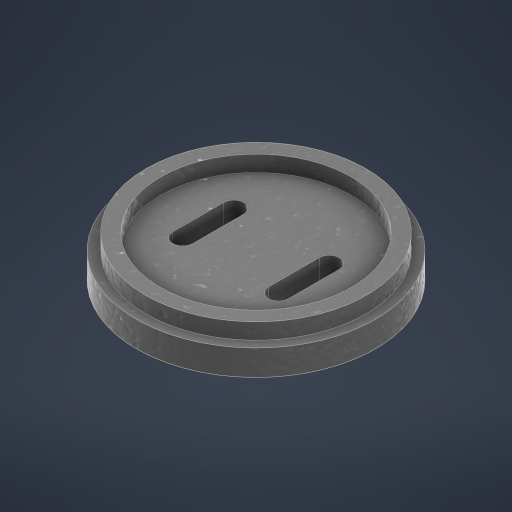
# Autodesk Inventor part: bay_bottom
Saved by Autodesk Inventor 2023 (Build 270158000, 158)
## iProperties
Created: 2022-11-18
Part Number: bay_bottom
Material: Generic
Document SubType Name: Modeling
Designer: washington
Density: 1 g/cm^3
Appearance: Fine Textured - Black
Author: washington
Autodesk Inventor part; units mm, degrees
ref_plane "YZ Plane" through (0, 0, 0) normal (1, 0, 0) x (0, 1, 0)
ref_plane "XZ Plane" through (0, 0, 0) normal (0, 1, 0) x (-1, 0, 0)
ref_plane "XY Plane" through (0, 0, 0) normal (0, 0, 1) x (1, 0, 0)
sketch "Sketch1" plane through (0, 0, 0) normal (0, 1, 0) x (-1, 0, 0)
  circle A0 centre (0, 0) radius 34.5
  circle A1 centre (0, 0) radius 37.5
  circle A2 centre (0, 0) radius 30
  line L0 (15, 8) -> (15, -8) construction
  line L1 (11.8377, 8) -> (11.8377, -8)
  line L2 (18.1623, -8) -> (18.1623, 8)
  arc A3 (18.1623, 8) -> (11.8377, 8) centre (15, 8) ccw
  arc A4 (11.8377, -8) -> (18.1623, -8) centre (15, -8) ccw
  line L3 (0, 16.7478) -> (0, 6) construction
  line L4 (-11.8377, 8) -> (-11.8377, -8)
  line L5 (-18.1623, -8) -> (-18.1623, 8)
  arc A5 (-11.8377, 8) -> (-18.1623, 8) centre (-15, 8) ccw
  arc A6 (-18.1623, -8) -> (-11.8377, -8) centre (-15, -8) ccw
  point P0 (15, 0)
  dimension "d0" = 69
  dimension "d1" = 75
  dimension "d2" = 60
  dimension "d3" = 15
  dimension "d4" = 16
  dimension "d5" = 8
  dimension "d6" = 3.1623
  dimension "d7" = 6
  dimension "d8" = 15
  dimension "d9" = 16.7478
  constraints: 14 end point, 8 point on circle, 7 centre point, 6 symmetric about line, 4 tangent, 3 coincident, 2 vertical, 1 midpoint, 1 parallel, 2 other
  measures "d0" diameter of A0
  measures "d1" diameter of A1
  measures "d2" diameter of A2
  measures "d3" distance of point (15, 0) point (0, 0)
  measures "d4" distance of L2.start L2.end
  measures "d5" vertical distance of point (0, 0) L0.end
  measures "d6" radius of A3
  measures "d7" distance of point (0, 0) L3.end
  measures "d8" distance between parallel lines of L3 L0
  measures "d9" distance of L3.start point (0, 0)
extrude "Extrusion1" add sketch "Sketch1" against normal blind 8 contours A0 | A1 | A2
extrude "Extrusion2" add sketch "Sketch1" along normal blind 5 contours A0
sketch "Sketch2" plane through (0, -8, 0) normal (0, -1, 0) x (1, 0, 0)
  line L0 (-5, 35) -> (5, 35)
  line L1 (5, 35) -> (5, -35)
  line L2 (5, -35) -> (-5, -35)
  line L3 (-5, -35) -> (-5, 35)
  line L4 (-5, 35) -> (5, -35) construction
  line L5 (5, 35) -> (-5, -35) construction
  point P0 (0, 0)
  point P1 (0, 35)
  dimension "d16" = 10
  dimension "d17" = 70
  constraints: 12 end point, 3 midpoint, 2 parallel, 1 horizontal, 1 perpendicular
  measures "d16" distance between parallel lines of L1 L3
  measures "d17" distance from line of point (0, 35) L2
extrude "Extrusion3" cut sketch "Sketch2" against normal blind 5
body "Solid1"
